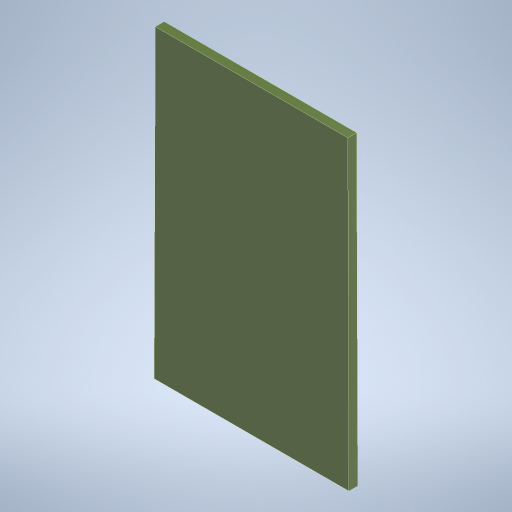
# Autodesk Inventor part: PCB-V1
Saved by Autodesk Inventor 2024.3 (Build 283343000, 343)
## iProperties
Created: 2025-01-22
Part Number: PCB-V1
Material: Copper
Document SubType Name: Modeling
Designer: ASUS TUF
Density: 8.94 g/cm^3
Appearance: Dark Olive
Author: ASUS TUF
Autodesk Inventor part; units mm, degrees
ref_plane "YZ Plane" through (0, 0, 0) normal (1, 0, 0) x (0, 1, 0)
ref_plane "XZ Plane" through (0, 0, 0) normal (0, 1, 0) x (-1, 0, 0)
ref_plane "XY Plane" through (0, 0, 0) normal (0, 0, 1) x (1, 0, 0)
sketch "Sketch1" plane through (0, 0, 0) normal (0, 0, 1) x (1, 0, 0)
  line L0 (-21.75, 34.4998) -> (21.75, 34.4998)
  line L1 (21.75, 34.4998) -> (22, -34.4998)
  line L2 (22, -34.4998) -> (-22, -34.4998)
  line L3 (-22, -34.4998) -> (-21.75, 34.4998)
  point P0 (0, 0)
  point P1 (0, 34.4998)
  point P2 (0, -34.4998)
  point P3 (21.875, 0)
  dimension "d0" = 43.5
  dimension "d1" = 69
  dimension "d2" = 44
  dimension "d3" = 69
  constraints: 8 end point, 3 midpoint, 2 vertical alignment, 1 horizontal, 1 horizontal alignment
  measures "d0" distance of L0.start L0.end
  measures "d1" distance of L0.end L1.end
  measures "d2" distance of L1.end L2.end
  measures "d3" distance of L0.start L2.end
extrude "Extrusion1" add sketch "Sketch1" along normal mid plane 2
body "Solid1"
